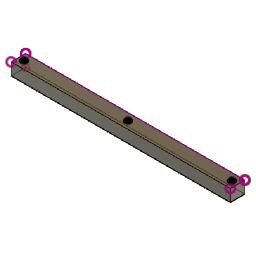
Rack (Autodesk Fusion 360 design; units mm, degrees)
Autodesk Fusion 360 part; units mm, degrees
sketch "Sketch1" plane through (0, 0, 0) normal (0, 0, 1) x (1, 0, 0)
  line L0 (0, 0) -> (180, 0)
  line L1 (180, 0) -> (180, -12)
  line L2 (180, -12) -> (0, -12)
  line L3 (0, -12) -> (0, 0)
  dimension "d16" = 180
  dimension "d17" = 12
  constraint horizontal L0
  constraint vertical L1
  constraint horizontal L2
  constraint vertical L3
  constraint coincident L0.start L3.end
  measures "d16" distance of L0.start L0.end
  measures "d17" distance of L0.start L2.end
extrude "Extrude1" add sketch "Sketch1" along normal blind 10
sketch "Sketch6" plane through (0, 0, 10) normal (0, 0, 1) x (-1, 0, 0)
  line L0 (0, 12) -> (-180, 12)
  line L1 (-180, 12) -> (-180, 0)
  line L2 (-180, 0) -> (0, 0)
  line L3 (0, 0) -> (0, 12)
  circle A0 centre (-4.7, 6) radius 1.5
  circle A1 centre (-4.7, 6) radius 2.7
  circle A2 centre (-175.3, 6) radius 1.5
  circle A3 centre (-175.3, 6) radius 2.7
  line L4 (0, 12) -> (0, 0)
  line L5 (0, 0) -> (-180, 0)
  line L6 (-180, 0) -> (-180, 12)
  circle A4 centre (-90, 6) radius 1.5
  circle A5 centre (-90, 6) radius 2.7
  dimension "d65" = 3
  dimension "d66" = 1.2
  dimension "d67" = 3
  dimension "d68" = 1.2
  dimension "d69" = 4.7
  dimension "d70" = 6
  dimension "d71" = 4.7
  dimension "d72" = 6
  dimension "d82" = 3
  dimension "d83" = 1.2
  dimension "d88" = 6
  dimension "d89" = 90
  measures "d65" diameter of A0
  measures "d67" diameter of A2
  measures "d69" distance of A0.centre L4
  measures "d70" distance of A0.centre L5
  measures "d71" distance of A2.centre L6
  measures "d72" distance of A2.centre L5
  measures "d82" diameter of A4
  measures "d88" distance of L5 A4.centre
  measures "d89" distance of L4 A4.centre
extrude "Extrude9" cut sketch "Sketch6" against normal blind 100 contours A2
extrude "Extrude10" cut sketch "Sketch6" against normal blind 4 contours A3
extrude "Extrude11" cut sketch "Sketch6" against normal blind 100 contours A0
extrude "Extrude12" cut sketch "Sketch6" against normal blind 4 contours A1
extrude "Extrude13" cut sketch "Sketch6" against normal blind 100 contours A4
extrude "Extrude14" cut sketch "Sketch6" against normal blind 4 contours A5
equation "length = 180 mm"
equation "height = 10 mm"
equation "width = 12 mm"
equation "d16 = length"
equation "d17 = width"
equation "d18 = height"
equation "extra = 100 mm"
equation "bearing_outer_radius = 2.7 mm"
equation "bearing_width = 4 mm"
equation "bearing_big_distance = 2 mm + bearing_outer_radius"
equation "bearing_small_distance = width / 2"
equation "bearing_inner_radius = 1.5 mm"
equation "d65 = bearing_inner_radius * 2"
equation "d66 = bearing_outer_radius - bearing_inner_radius"
equation "d67 = bearing_inner_radius * 2"
equation "d68 = bearing_outer_radius - bearing_inner_radius"
equation "d69 = bearing_big_distance"
equation "d70 = bearing_small_distance"
equation "d71 = bearing_big_distance"
equation "d72 = bearing_small_distance"
equation "d73 = -extra"
equation "d75 = -bearing_width"
equation "d77 = -extra"
equation "d79 = -bearing_width"
equation "bearing_main_big_distance = length / 2"
equation "d82 = bearing_inner_radius * 2"
equation "d83 = bearing_outer_radius - bearing_inner_radius"
equation "d84 = -extra"
equation "d86 = -bearing_width"
equation "d88 = bearing_small_distance"
equation "d89 = bearing_main_big_distance"
